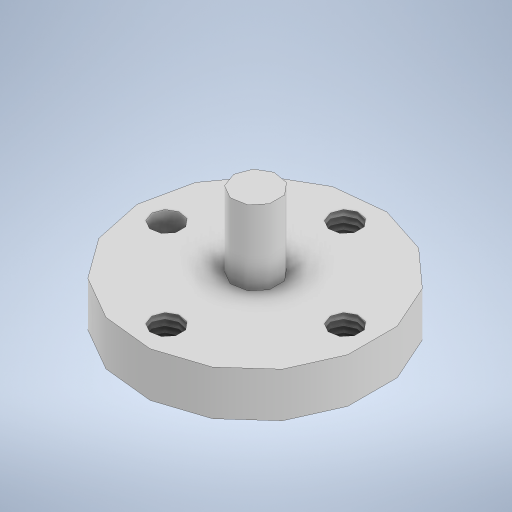
# Autodesk Inventor part: крутящаяся передача
Saved by Autodesk Inventor 2024.2 (Build 282272000, 272)
## iProperties
Created: 2025-11-25
Part Number: крутящаяся передача
Material: Типовые
Document SubType Name: Modeling
Designer: Zakhar
Density: 1 g/cm^3
Appearance: По умолчанию
Author: Zakhar
Autodesk Inventor part; units mm, degrees
ref_plane "YZ Plane" through (0, 0, 0) normal (1, 0, 0) x (0, 1, 0)
ref_plane "XZ Plane" through (0, 0, 0) normal (0, 1, 0) x (-1, 0, 0)
ref_plane "XY Plane" through (0, 0, 0) normal (0, 0, 1) x (1, 0, 0)
sketch "Эскиз1" plane through (0, 0, 0) normal (0, 1, 0) x (-1, 0, 0)
  circle A0 centre (0, 0) radius 8
  circle A1 centre (0, 6) radius 1
  circle A2 centre (-6, 0) radius 1
  circle A3 centre (0, -6) radius 1
  circle A4 centre (6, 0) radius 1
  circle A5 centre (0, 0) radius 1.5
  dimension "d0" = 16
  dimension "d1" = 2
  dimension "d2" = 6
  dimension "d5" = 360
  dimension "d7" = 3
  constraints: 6 centre point, 2 coincident, 9 other
  measures "d0" diameter of A0
  measures "d1" diameter of A1
  measures "d2" distance of point (0, 0) A1.centre
  measures "d7" diameter of A5
extrude "Выдавливание1" add sketch "Эскиз1" along normal blind 3
extrude "Выдавливание2" add sketch "Эскиз1" along normal blind 8 contours A5
thread "Резьба1" size "M2x0.4" class "6H" standard "ANSI Metric M Profile" full length
thread "Резьба2" size "M2x0.4" class "6H" standard "ANSI Metric M Profile" full length
thread "Резьба3" size "M2x0.4" class "6H" standard "ANSI Metric M Profile" full length
